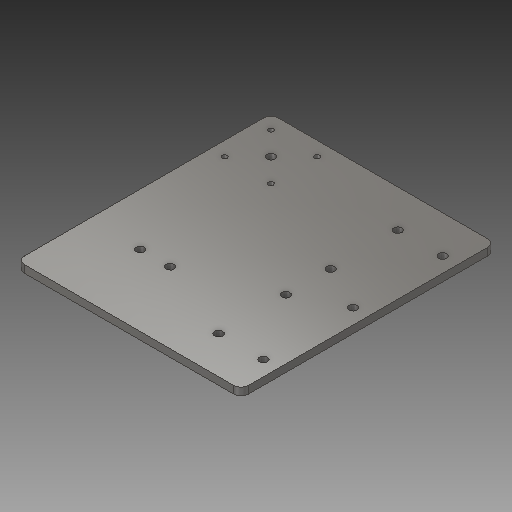
# Autodesk Inventor part: HeadPlate
Saved by Autodesk Inventor 2017 (Build 210142000, 142)
## iProperties
Created: 2016-12-13
Part Number: HeadPlate
Material: Steel, Carbon
Document SubType Name: Modeling
Designer: umr
Density: 7.85 g/cm^3
Appearance: Semi-Polished
Mass: 989.197 g
Surface Area: 546.459 cm^2
Volume: 126.012 cm^3
Author: umr
Autodesk Inventor part; units mm, degrees
ref_plane "YZ Plane" through (0, 0, 0) normal (1, 0, 0) x (0, 1, 0)
ref_plane "XZ Plane" through (0, 0, 0) normal (0, 1, 0) x (-1, 0, 0)
ref_plane "XY Plane" through (0, 0, 0) normal (0, 0, 1) x (1, 0, 0)
sketch "Sketch1" plane through (0, 0, 0) normal (0, 1, 0) x (-1, 0, 0)
  line L0 (0, 0) -> (150, 0)
  line L1 (150, 0) -> (150, -170)
  line L2 (150, -170) -> (0, -170)
  line L3 (0, -170) -> (0, 0)
  dimension "d0" = 150
  dimension "d1" = 170
  constraints: 8 end point, 2 parallel, 1 horizontal, 1 perpendicular
  measures "d0" distance of L1.end L2.end
  measures "d1" distance of L0.end L1.end
extrude "Extrusion1" add sketch "Sketch1" along normal blind 5
fillet "Fillet1" radius 5 4 edges at (0, 2.5, 0) (0, 2.5, -170) (-150, 2.5, 0) (-150, 2.5, -170)
sketch "Sketch2" plane through (0, 5, 0) normal (0, 1, 0) x (1, 0, 0)
  arc A0 (-145, 170) -> (-150, 165) centre (-145, 165) ccw projected
  line L0 (-150, 165) -> (-150, 5) projected
  arc A1 (-150, 5) -> (-145, 0) centre (-145, 5) ccw projected
  line L1 (-145, 0) -> (-5, 0) projected
  arc A2 (-5, 0) -> (0, 5) centre (-5, 5) ccw projected
  line L2 (0, 5) -> (0, 165) projected
  arc A3 (0, 165) -> (-5, 170) centre (-5, 165) ccw projected
  line L3 (-5, 170) -> (-145, 170) projected
  circle A4 centre (-125, 145) radius 2.75
  circle A5 centre (-140.5, 160.5) radius 1.75
  circle A6 centre (-140.5, 129.5) radius 1.75
  circle A7 centre (-109.5, 160.5) radius 1.75
  circle A8 centre (-109.5, 129.5) radius 1.75
  circle A9 centre (-40, 25) radius 2.75
  circle A10 centre (-10, 25) radius 2.75
  circle A11 centre (-40, 145) radius 2.75
  circle A12 centre (-10, 145) radius 2.75
  circle A13 centre (-10, 85) radius 2.75
  circle A14 centre (-40, 70) radius 2.75
  circle A15 centre (-40, 100) radius 2.75
  circle A16 centre (-115, 47.5) radius 2.75
  circle A17 centre (-95, 47.5) radius 2.75
  point P0 (0, 0)
  dimension "d5" = 5.5
  dimension "d6" = 25
  dimension "d7" = 25
  dimension "d8" = 3.5
  dimension "d9" = 9.5
  dimension "d10" = 9.5
  dimension "d13" = 31
  dimension "d16" = 31
  dimension "d19" = 5.5
  dimension "d20" = 25
  dimension "d21" = 5.5
  dimension "d22" = 25
  dimension "d23" = 5.5
  dimension "d24" = 5.5
  dimension "d25" = 25
  dimension "d26" = 25
  dimension "d27" = 5.5
  dimension "d28" = 170
  dimension "d29" = 85
  dimension "d30" = 5.5
  dimension "d31" = 5.5
  dimension "d32" = 30
  dimension "d33" = 70
  dimension "d34" = 10
  dimension "d35" = 10
  dimension "d36" = 10
  dimension "d37" = 40
  dimension "d38" = 40
  dimension "d39" = 40
  dimension "d40" = 40
  dimension "d43" = 5.5
  dimension "d44" = 5.5
  dimension "d45" = 45
  dimension "d46" = 22.5
  dimension "d47" = 22.5
  dimension "d48" = 20
  dimension "d49" = 35
  constraints: 14 centre point, 1 horizontal, 1 vertical, 6 other
  measures "d5" diameter of A4
  measures "d6" distance from line of L3 A4.centre
  measures "d7" distance from line of L0 A4.centre
  measures "d8" diameter of A5
  measures "d9" distance from line of A5.centre L3
  measures "d10" distance from line of L0 A5.centre
  measures "d13" distance of A5.centre A6.centre
  measures "d16" distance of A5.centre A7.centre
  measures "d19" diameter of A9
  measures "d20" distance from line of L1 A9.centre
  measures "d21" diameter of A10
  measures "d22" distance from line of L1 A10.centre
  measures "d23" diameter of A11
  measures "d24" diameter of A12
  measures "d25" distance from line of L3 A11.centre
  measures "d26" distance from line of L3 A12.centre
  measures "d27" diameter of A13
  measures "d28" distance between parallel lines of L3 L1
  measures "d29" distance from line of L3 A13.centre
  measures "d30" diameter of A14
  measures "d31" diameter of A15
  measures "d32" distance of A15.centre A14.centre
  measures "d33" distance from line of L3 A15.centre
  measures "d34" distance from line of L2 A10.centre
  measures "d35" distance from line of L2 A13.centre
  measures "d36" distance from line of L2 A12.centre
  measures "d37" distance from line of L2 A9.centre
  measures "d38" distance from line of L2 A14.centre
  measures "d39" distance from line of L2 A15.centre
  measures "d40" distance from line of L2 A11.centre
  measures "d43" diameter of A16
  measures "d44" diameter of A17
  measures "d45" distance of A9.centre A14.centre
  measures "d46" vertical distance of A14.centre A16.centre
  measures "d47" vertical distance of A14.centre A17.centre
  measures "d48" distance of A16.centre A17.centre
  measures "d49" distance from line of L0 A16.centre
extrude "Extrusion2" cut sketch "Sketch2" against normal blind 5 contours A4 | A5 | A6 | A7 | A8 | A9 | A10 | A11 | A12 | A13 | A14 | A15 | A16 | A17
equation "\"d20\" = d6"
equation "\"d22\" = d20"
equation "\"d25\" = d6"
equation "\"d26\" = d25"
equation "\"d29\" = 0.5 * d28"
equation "\"d33\" = 0.5 * d28 - 0.5 * d32"
equation "\"d35\" = d34"
equation "\"d36\" = d34"
equation "\"d38\" = d37"
equation "\"d39\" = d38"
equation "\"d40\" = d37"
equation "\"d46\" = 0.5 * d45"
equation "\"d47\" = d46"
body "Solid1"
